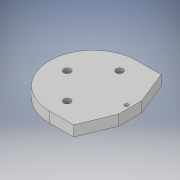
# Autodesk Inventor part: 000.403 -  Прижим подшипников
Saved by Autodesk Inventor 2019 (Build 230136000, 136)
## iProperties
Created: 2020-03-23
Part Number: 000.403 -  Прижим подшипников
Material: Типовые
Document SubType Name: Modeling
Designer: Петров Иван
Density: 1 g/cm^3
Appearance: По умолчанию
Author: Петров Иван
Autodesk Inventor part; units mm, degrees
ref_plane "YZ Plane" through (0, 0, 0) normal (1, 0, 0) x (0, 1, 0)
ref_plane "XZ Plane" through (0, 0, 0) normal (0, 1, 0) x (-1, 0, 0)
ref_plane "XY Plane" through (0, 0, 0) normal (0, 0, 1) x (1, 0, 0)
sketch "Эскиз1" plane through (0, 0, 0) normal (0, 1, 0) x (-1, 0, 0)
  circle A0 centre (15.0247, -0.005) radius 9.5
  circle A1 centre (0.0247, 14.995) radius 9.5
  circle A2 centre (0.0247, -15.005) radius 9.5
  arc A3 (-4.923, -24.5094) -> (-4.9258, 24.5) centre (0.0275, -0.0044) ccw
  arc A4 (-13.7779, 22.8932) -> (-4.9258, 24.5) centre (-49.9753, 247.495) ccw
  line L0 (-13.7779, 22.8932) -> (-13.7779, -22.9031)
  arc A5 (-4.923, -24.5094) -> (-4.9258, 24.5) centre (0.0275, -0.0044) ccw
  circle A6 centre (15.0247, -0.005) radius 9.5
  circle A7 centre (0.0247, 14.995) radius 9.5
  circle A8 centre (0.0247, -15.005) radius 9.5
  arc A9 (-4.923, -24.5094) -> (-4.9258, 24.5) centre (0.0275, -0.0044) ccw
  arc A10 (-13.7779, 22.8932) -> (-4.9258, 24.5) centre (-49.9753, 247.495) ccw
  arc A11 (-4.923, -24.5094) -> (-13.7779, -22.9031) centre (-49.9479, -247.5094) ccw
  line L1 (-13.7779, 22.8932) -> (-13.7779, -22.9031)
  arc A12 (-4.923, -24.5094) -> (-4.9258, 24.5) centre (0.0275, -0.0044) ccw
  line L2 (0.0275, -25.0044) -> (-13.7779, -25.0044)
  line L3 (-13.7779, -25.0044) -> (-13.7779, -22.9031)
  line L4 (0.0275, 24.9956) -> (-13.7779, 24.9956)
  line L5 (-13.7779, 24.9956) -> (-13.7779, 22.8932)
  point P0 (0, 0)
  constraints: 19 point on circle, 13 centre point, 12 end point, 8 tangent, 2 coincident, 2 concentric, 2 horizontal, 2 perpendicular, 2 vertical
extrude "Выдавливание1" add sketch "Эскиз1" along normal blind 6 contours A0 | A1 | A2 | A11 L0 A4 A3 | A3 L2 L3 A11 | A3 A4 L5 L4
sketch "Эскиз3" plane through (0, 6, 0) normal (0, 1, 0) x (1, 0, 0)
  line L0 (13.7779, -24.9956) -> (13.7779, 25.0044) projected
  line L1 (13.7779, 25.0044) -> (-0.0275, 25.0044) projected
  arc A0 (-0.0275, 25.0044) -> (-0.0275, -24.9956) centre (-0.0275, 0.0044) ccw projected
  line L2 (-0.0275, -24.9956) -> (13.7779, -24.9956) projected
  point P0 (0, 0)
sketch "Эскиз4" plane through (0, 6, 0) normal (0, 1, 0) x (1, 0, 0)
  circle A0 centre (-14.9698, -0.0039) radius 9.5
  circle A1 centre (0.0302, -15.0039) radius 9.5
  circle A2 centre (0.0302, 14.9961) radius 9.5
  arc A3 (4.9779, 24.5005) -> (4.9807, -24.5088) centre (0.0275, -0.0044) ccw
  arc A4 (13.8328, -22.902) -> (4.9807, -24.5088) centre (50.0302, -247.5039) ccw
  line L0 (13.8328, -22.902) -> (13.8328, 22.8943)
  arc A5 (4.9779, 24.5005) -> (4.9807, -24.5088) centre (0.0275, -0.0044) ccw
  circle A6 centre (-14.9698, -0.0039) radius 9.5
  circle A7 centre (0.0302, -15.0039) radius 9.5
  circle A8 centre (0.0302, 14.9961) radius 9.5
  arc A9 (4.9779, 24.5005) -> (4.9807, -24.5088) centre (0.0275, -0.0044) ccw
  arc A10 (13.8328, -22.902) -> (4.9807, -24.5088) centre (50.0302, -247.5039) ccw
  arc A11 (4.9779, 24.5005) -> (13.8328, 22.8943) centre (50.0028, 247.5006) ccw
  line L1 (13.8328, -22.902) -> (13.8328, 22.8943)
  arc A12 (4.9779, 24.5005) -> (4.9807, -24.5088) centre (0.0275, -0.0044) ccw
  line L2 (0.0275, 24.9956) -> (13.8328, 24.9956)
  line L3 (13.8328, 24.9956) -> (13.8328, 22.8943)
  line L4 (0.0275, -25.0044) -> (13.8328, -25.0044)
  line L5 (13.8328, -25.0044) -> (13.8328, -22.902)
  circle A13 centre (-14.9698, -0.0039) radius 2
  circle A14 centre (0.0302, 14.9961) radius 2
  circle A15 centre (0.0302, -15.0039) radius 2
  point P0 (0, 0)
  point P1 (0.0549, -0.0088)
  dimension "d12" = 4
  dimension "d13" = 4
  dimension "d14" = 4
  constraints: 19 point on circle, 16 centre point, 12 end point, 8 tangent, 5 coincident, 2 concentric, 2 perpendicular
  measures "d12" diameter of A13
  measures "d13" diameter of A14
  measures "d14" diameter of A15
extrude "Выдавливание3" cut sketch "Эскиз4" against normal blind 10 contours A13 | A14 | A15
sketch "Эскиз5" plane through (0, 0, 0) normal (0, -1, 0) x (1, 0, 0)
  circle A0 centre (0.0302, 15.0039) radius 2 projected
  circle A1 centre (0.0302, 15.0039) radius 4
  circle A2 centre (-14.9698, 0.0039) radius 2 projected
  circle A3 centre (-14.9698, 0.0039) radius 4
  circle A4 centre (0.0302, -14.9961) radius 2 projected
  circle A5 centre (0.0302, -14.9961) radius 4
  point P0 (0, 0)
  dimension "d17" = 8
  dimension "d18" = 8
  dimension "d19" = 8
  constraints: 3 centre point, 3 coincident
  measures "d17" diameter of A1
  measures "d18" diameter of A3
  measures "d19" diameter of A5
extrude "Выдавливание4" cut sketch "Эскиз5" against normal blind 3
sketch "Эскиз6" plane through (0, 0, 0) normal (0, -1, 0) x (1, 0, 0)
  line L0 (5.48, 2.9) -> (5.6, 2.9)
  arc A0 (5.6, -2.9) -> (5.6, 2.9) centre (5.6, 0) ccw
  line L1 (5.6, -2.9) -> (5.48, -2.9)
  arc A1 (1.562, -6) -> (5.48, -2.9) centre (0, 0) ccw
  line L2 (1.562, -6) -> (15.55, -6)
  arc A2 (15.55, -6) -> (16.3, -5.25) centre (15.55, -5.25) ccw
  line L3 (16.3, -5.25) -> (16.3, 5.25)
  arc A3 (16.3, 5.25) -> (15.55, 6) centre (15.55, 5.25) ccw
  line L4 (15.55, 6) -> (1.562, 6)
  arc A4 (5.48, 2.9) -> (1.562, 6) centre (0, 0) ccw
  line L5 (9.9, -5.1) -> (14.9, -5.1)
  arc A5 (9.4, -4.6) -> (9.9, -5.1) centre (9.9, -4.6) ccw
  line L6 (9.4, 4.6) -> (9.4, -4.6)
  arc A6 (9.9, 5.1) -> (9.4, 4.6) centre (9.9, 4.6) ccw
  line L7 (14.9, 5.1) -> (9.9, 5.1)
  arc A7 (15.4, 4.6) -> (14.9, 5.1) centre (14.9, 4.6) ccw
  line L8 (15.4, -4.6) -> (15.4, 4.6)
  arc A8 (14.9, -5.1) -> (15.4, -4.6) centre (14.9, -4.6) ccw
  arc A9 (20.0026, 0.55) -> (20.0026, -0.55) centre (19.05, 0) ccw
  line L9 (21.2, 0.55) -> (20.0026, 0.55)
  line L10 (21.2, 0.55) -> (21.2, 5.25)
  arc A10 (21.2, 5.25) -> (20.35, 6.1) centre (20.35, 5.25) ccw
  line L11 (20.35, 6.1) -> (15.55, 6.1)
  arc A11 (16.4, 5.25) -> (15.55, 6.1) centre (15.55, 5.25) ccw
  line L12 (16.4, -5.25) -> (16.4, 5.25)
  arc A12 (15.55, -6.1) -> (16.4, -5.25) centre (15.55, -5.25) ccw
  line L13 (15.55, -6.1) -> (20.35, -6.1)
  arc A13 (20.35, -6.1) -> (21.2, -5.25) centre (20.35, -5.25) ccw
  line L14 (21.2, -5.25) -> (21.2, -0.55)
  line L15 (20.0026, -0.55) -> (21.2, -0.55)
  line L16 (-10.9, 5.25) -> (-10.9, 0.55)
  line L17 (-9.7026, 0.55) -> (-10.9, 0.55)
  arc A14 (-9.7026, -0.55) -> (-9.7026, 0.55) centre (-8.75, 0) ccw
  line L18 (-10.9, -0.55) -> (-9.7026, -0.55)
  line L19 (-10.9, -0.55) -> (-10.9, -5.25)
  arc A15 (-10.9, -5.25) -> (-10.05, -6.1) centre (-10.05, -5.25) ccw
  line L20 (-10.05, -6.1) -> (-5.25, -6.1)
  arc A16 (-6.1, -5.25) -> (-5.25, -6.1) centre (-5.25, -5.25) ccw
  line L21 (-6.1, 5.25) -> (-6.1, -5.25)
  arc A17 (-5.25, 6.1) -> (-6.1, 5.25) centre (-5.25, 5.25) ccw
  line L22 (-5.25, 6.1) -> (-10.05, 6.1)
  arc A18 (-10.05, 6.1) -> (-10.9, 5.25) centre (-10.05, 5.25) ccw
  line L23 (-5.25, 6.1) -> (-1.562, 6.1)
  line L24 (1.562, 6.1) -> (0, 6.1)
  line L25 (0, 6.1) -> (-1.562, 6.1)
  line L26 (1.562, 6.1) -> (15.55, 6.1)
  line L27 (15.55, -6.1) -> (1.562, -6.1)
  line L28 (-1.562, -6.1) -> (-5.25, -6.1)
  line L29 (-1.562, -6.1) -> (0, -6.1)
  line L30 (0, -6.1) -> (1.562, -6.1)
  arc A19 (-1.562, 6) -> (-6, 1.562) centre (0, 0) ccw
  line L31 (-1.562, 6) -> (-5.25, 6)
  arc A20 (-5.25, 6) -> (-6, 5.25) centre (-5.25, 5.25) ccw
  line L32 (-6, 5.25) -> (-6, 1.562)
  line L33 (-5.25, -6) -> (-1.562, -6)
  arc A21 (-6, -1.562) -> (-1.562, -6) centre (0, 0) ccw
  line L34 (-6, -1.562) -> (-6, -5.25)
  arc A22 (-6, -5.25) -> (-5.25, -6) centre (-5.25, -5.25) ccw
  circle A23 centre (19.05, 0) radius 1.1
  line L35 (20.0026, 0.55) -> (21.2, 0.55)
  line L36 (21.2, -0.55) -> (21.2, 0.55)
  circle A24 centre (-8.75, 0) radius 1.1
  line L37 (-10.9, 0.55) -> (-9.7026, 0.55)
  line L38 (-10.9, -0.55) -> (-10.9, 0.55)
  circle A25 centre (0, 0) radius 0.8
  line L39 (21.2, 5.25) -> (21.2, 6.6315)
  line L40 (-0.0275, 24.9956) -> (13.7779, 24.9956) projected
  line L41 (21.2, 6.6315) -> (13.7779, 24.9956)
  line L42 (19.05, 0) -> (20.0026, 0)
  line L43 (21.2, -5.25) -> (21.2, -6.6315)
  line L44 (21.2, -6.6315) -> (13.7779, -24.9956)
  line L45 (13.7779, -24.9956) -> (13.7779, 24.9956)
  line L46 (13.7779, -25.0044) -> (-0.0275, -25.0044) projected
  point P0 (5.15, 0)
  constraints: 90 end point, 46 point on circle, 25 centre point, 2 coincident, 2 symmetric about line, 2 vertical, 1 collinear, 1 concentric, 1 horizontal, 1 perpendicular, 1 tangent, 3 other
extrude "Выдавливание5" add sketch "Эскиз6" against normal blind 6 contours L45 L26 A11 L12 A12 L27 L2 A2 L3 A3 L4 | L4 A3 L3 A2 L2 L45 L5 A8 L8 A7 L7 | L7 A7 L8 A8 L5 L45 | L45 L41 L39 A10 L11 L26 | L11 A10 L10 L9 A9 L15 L14 A13 L13 A12 L12 A11 | L27 L13 A13 L43 L44 L45 | L36 L15 A23 L9
